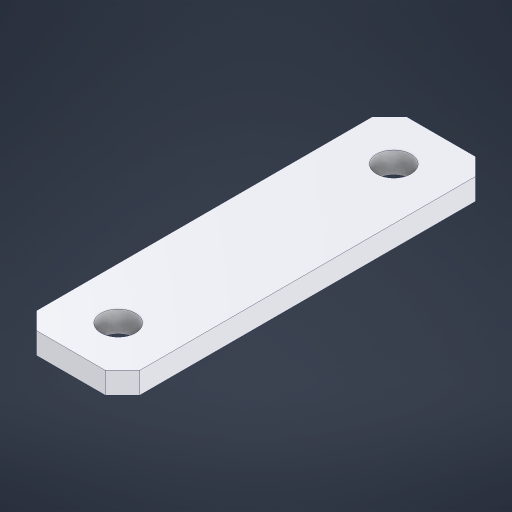
# Autodesk Inventor part: ArmMotorSpacer
Saved by Autodesk Inventor 2024 (Build 280153000, 153)
## iProperties
Created: 2023-10-20
Part Number: ArmMotorSpacer
Material: Generic
Document SubType Name: Modeling
Designer: avsar
Density: 1 g/cm^3
Appearance: PTFE
Author: avsar
Autodesk Inventor part; units mm, degrees
ref_plane "YZ Plane" through (0, 0, 0) normal (1, 0, 0) x (0, 1, 0)
ref_plane "XZ Plane" through (0, 0, 0) normal (0, 1, 0) x (-1, 0, 0)
ref_plane "XY Plane" through (0, 0, 0) normal (0, 0, 1) x (1, 0, 0)
sketch "Sketch1" plane through (0, 0, 0) normal (0, 1, 0) x (-1, 0, 0)
  line L0 (-6, 21.5) -> (6, 21.5)
  line L1 (6, 21.5) -> (6, -21.5)
  line L2 (6, -21.5) -> (-6, -21.5)
  line L3 (-6, -21.5) -> (-6, 21.5)
  line L4 (-6, 21.5) -> (6, -21.5) construction
  line L5 (6, 21.5) -> (-6, -21.5) construction
  point P0 (0, 0)
  dimension "d0" = 12
  dimension "d1" = 43
  constraints: 12 end point, 2 midpoint, 2 parallel, 1 horizontal, 1 perpendicular
  measures "d0" distance of L1.end L2.end
  measures "d1" distance of L0.end L1.end
extrude "Extrusion1" add sketch "Sketch1" along normal mid plane 2.5
sketch "Sketch2" plane through (0, 1.25, 0) normal (0, 1, 0) x (1, 0, 0)
  circle A0 centre (0, -16) radius 2
  line L0 (6, 21.5) -> (-6, 21.5) construction
  line L1 (-6, 21.5) -> (-6, -21.5) construction
  line L2 (-6, -21.5) -> (6, -21.5) construction
  line L3 (6, -21.5) -> (6, 21.5) construction
  line L4 (-6, 21.5) -> (-6, -21.5) construction
  line L5 (-6, 0) -> (6, 0) construction
  circle A1 centre (0, 16) radius 2
  point P0 (0, 0)
  dimension "d4" = 4
  dimension "d5" = 16
  constraints: 2 centre point, 2 end point, 2 midpoint, 1 symmetric about line, 1 vertical alignment, 1 other
  measures "d4" diameter of A0
  measures "d5" distance of point (0, 0) A0.centre
extrude "Extrusion2" cut sketch "Sketch2" against normal through all
chamfer "Chamfer1" distance 2 angle 45 4 edges at (-6, 0, 21.5) (6, 0, 21.5) (6, 0, -21.5) (-6, 0, -21.5)
body "Solid1"
